Autodesk Fusion 360 part; units mm, degrees
note: some values were not read from the file. Chosen so that the rebuilt part matches the saved one: which bodies a step acts on; which face or edge a step refers to; where a step ends.
(part 2 of 2)
sketch "Sketch2 (3)" plane through (-245, 0, 0) normal (-1, 0, 0) x (0, 0, 1) in component "Обшивка-Плиты"
  line L0 (-212.9492, 20) -> (-218.3368, 15)
  line L1 (-218.3368, 15) -> (0, 15)
  line L2 (0, 15) -> (0, 20)
  line L3 (0, 20) -> (-212.9492, 20)
  line L4 (-500, 15) -> (-250, 15)
  line L5 (-250, 15) -> (-250, 140)
  line L6 (-250, 140) -> (-500, 140)
  line L7 (-500, 140) -> (-500, 15)
  line L8 (-500, 140) -> (-250, 140)
  line L9 (-250, 140) -> (-250, 265)
  line L10 (-250, 265) -> (-500, 265)
  line L11 (-500, 265) -> (-500, 140)
  line L12 (-250, 15) -> (0, 15)
  line L13 (0, 15) -> (0, 140)
  line L14 (0, 140) -> (-250, 140)
  line L15 (-250, 140) -> (-250, 15)
  line L16 (-250, 140) -> (0, 140)
  line L17 (0, 140) -> (0, 265)
  line L18 (0, 265) -> (-250, 265)
  line L19 (-250, 265) -> (-250, 140)
  point P0 (-500, 15)
  dimension "d244" = 250
  dimension "d245" = 125
  dimension "d246" = 250
  dimension "d247" = 125
  dimension "d248" = 250
  dimension "d249" = 125
  dimension "d250" = 250
  dimension "d251" = 125
  constraint horizontal L4
  constraint vertical L5
  constraint horizontal L6
  constraint vertical L7
  constraint coincident P0 L4.start
  constraint horizontal L8
  constraint vertical L9
  constraint horizontal L10
  constraint vertical L11
  constraint horizontal L12
  constraint vertical L13
  constraint horizontal L14
  constraint vertical L15
  constraint horizontal L16
  constraint vertical L17
  constraint horizontal L18
  constraint vertical L19
  measures "d244" distance of P0 L4.end
  measures "d245" distance of P0 L6.end
  measures "d246" distance of L6.end L5.end
  measures "d247" distance of L6.end L10.end
  measures "d248" distance of L4.end L1.end
  measures "d249" distance of L4.end L5.end
  measures "d250" distance of L5.end L13.end
  measures "d251" distance of L5.end L9.end
extrude "Extrude6''" add sketch "Sketch2 (3)" along normal blind 1.12 separate body contours L4 L5 L6 L7 L8 L15 makes body 113 in component "Обшивка-Плиты"
extrude "Extrude7" add sketch "Sketch2 (3)" along normal blind 1.12 separate body contours L6 L8 L9 L10 L11 L19 makes body 114 in component "Обшивка-Плиты"
extrude "Extrude8" add sketch "Sketch2 (3)" along normal blind 1.12 separate body contours L9 L14 L16 L17 L18 L19 makes body 115 in component "Обшивка-Плиты"
extrude "Extrude9" add sketch "Sketch2 (3)" along normal blind 1.12 separate body contours L0 L1 L2 L3 L12 L13 | L0 L3 L5 L12 L13 L14 L15 L16 makes body 116 in component "Обшивка-Плиты"
split "Split1" by plane through (-259.4882, 213.5887, -495) normal (-0.190809, 0.981627, 0) bodies 114 115 makes body 118 at (-246.12, 232.4581, -83.3333) makes body 117 at (-246.12, 232.4581, -333.3333) in component "Обшивка-Плиты"
delete_body "RemoveBody1" bodies 118 in component "Обшивка-Плиты"
delete_body "RemoveBody2" bodies 117 in component "Обшивка-Плиты"
combine "Combine5'" operation cut target body 114 tool bodies 79 78 77 76 75 keep tools in component "Обшивка-Плиты"
combine "Combine6'" operation cut target body 115 tool bodies 74 73 72 71 keep tools in component "Обшивка-Плиты"
sketch "Sketch3 (3)" plane through (0, 0, 0) normal (0, 0, 1) x (1, 0, 0) in component "Обшивка-Плиты"
  line L0 (-194.3541, 20) -> (-199.0829, 15)
  line L1 (-199.0829, 15) -> (-5, 15)
  line L2 (-5, 15) -> (-5, 20)
  line L3 (-5, 20) -> (-194.3541, 20)
  line L4 (-245, 15) -> (5, 15)
  line L5 (5, 15) -> (5, 140)
  line L6 (5, 140) -> (-245, 140)
  line L7 (-245, 140) -> (-245, 15)
  line L8 (-245, 140) -> (5, 140)
  line L9 (5, 140) -> (5, 265)
  line L10 (5, 265) -> (-245, 265)
  line L11 (-245, 265) -> (-245, 140)
  point P0 (-245, 15)
  dimension "d260" = 250
  dimension "d261" = 125
  dimension "d262" = 250
  dimension "d263" = 125
  constraint horizontal L4
  constraint vertical L5
  constraint horizontal L6
  constraint vertical L7
  constraint coincident P0 L4.start
  constraint horizontal L8
  constraint vertical L9
  constraint horizontal L10
  constraint vertical L11
  measures "d260" distance of P0 L4.end
  measures "d261" distance of P0 L6.end
  measures "d262" distance of L6.end L5.end
  measures "d263" distance of L6.end L10.end
extrude "Extrude10" add sketch "Sketch3 (3)" along normal blind 1.12 separate body contours L0 L1 L2 L3 L4 | L0 L2 L3 L4 L5 L6 L7 L8 makes body 119 in component "Обшивка-Плиты"
extrude "Extrude11" add sketch "Sketch3 (3)" along normal blind 1.12 separate body contours L6 L8 L9 L10 L11 makes body 120 in component "Обшивка-Плиты"
split "Split2" by plane through (-259.4882, 213.5887, 0) normal (-0.190809, 0.981627, 0) bodies 120 makes body 121 at (-161.6667, 248.8016, 0) in component "Обшивка-Плиты"
delete_body "RemoveBody3" bodies 121 in component "Обшивка-Плиты"
mirror "Mirror1" about plane through (0, 0, -250) normal (0, 0, 1) of bodies 119 120 makes body 122 at (-146.361, 98.3333, -500) makes body 123 at (-78.3333, 207.135, -500) in component "Обшивка-Плиты"
extrude "Extrude12" add sketch "Sketch1 (9)" along normal blind 1.12 separate body contours L5 L13 L16 L17 L18 L19 makes body 124 in component "Обшивка-Плиты"
combine "Combine7'" operation cut target body 124 tool bodies 74 keep tools in component "Обшивка-Плиты"
sketch "Sketch1 (10)" plane through (5, 0, 0) normal (1, 0, 0) x (0, 0, -1) in component "Обшивка-Доски"
  line L0 (270.8891, 15) -> (275, 20)
  line L1 (275, 20) -> (0, 20)
  line L2 (0, 20) -> (0, 15)
  line L3 (0, 15) -> (270.8891, 15)
  line L4 (0, 15) -> (125, 15)
  line L5 (125, 15) -> (125, 30)
  line L6 (125, 30) -> (0, 30)
  line L7 (0, 30) -> (0, 15)
  point P0 (0, 15)
  dimension "d273" = 125
  dimension "d274" = 15
  constraint horizontal L4
  constraint vertical L5
  constraint horizontal L6
  constraint vertical L7
  constraint coincident P0 L2.end
  measures "d273" distance of P0 L4.end
  measures "d274" distance of P0 L6.end
extrude "Extrude1'''''''''" add sketch "Sketch1 (10)" along normal blind 1 separate body contours L1 L2 L3 L4 L5 L7 | L1 L5 L6 L7 makes body 125 in component "Обшивка-Доски"
pattern_linear "R-Pattern1''''''" count 17 spacing 15 along (0, 1, 0) of bodies 125 makes body 126 at (5, 38.3333, -41.6667) makes body 127 at (5, 53.3333, -41.6667) makes body 128 at (5, 68.3333, -41.6667) makes body 129 at (5, 83.3333, -41.6667) makes body 130 at (5, 98.3333, -41.6667) makes body 131 at (5, 113.3333, -41.6667) makes body 132 at (5, 128.3333, -41.6667) makes body 133 at (5, 143.3333, -41.6667) makes body 134 at (5, 158.3333, -41.6667) makes body 135 at (5, 173.3333, -41.6667) makes body 136 at (5, 188.3333, -41.6667) makes body 137 at (5, 203.3333, -41.6667) makes body 138 at (5, 218.3333, -41.6667) makes body 139 at (5, 233.3333, -41.6667) makes body 140 at (5, 248.3333, -41.6667) makes body 141 at (5, 263.3333, -41.6667) in component "Обшивка-Доски"
split "Split1'" by plane through (230.3104, 308.7959, 0) normal (0.190809, -0.981627, 0) bodies 141 makes body 142 at (6, 263.4629, -41.6667) in component "Обшивка-Доски"
delete_body "RemoveBody1'" bodies 141 in component "Обшивка-Доски"
copy_body "CopyPasteBodies1'''''" bodies 138 139 140 142 makes body 143 makes body 144 makes body 145 makes body 146
move_body "Move1'''''''" bodies 143 144 145 146 to x (1, 0, 0) y (0, 1, 0) z (0, 0, 1) at (0, 0, -125)
delete_body "RemoveBody1''" bodies 143
delete_body "RemoveBody2'" bodies 146
delete_body "RemoveBody3'" bodies 145
delete_body "RemoveBody4'" bodies 144
copy_body "CopyPasteBodies1''''''" bodies 142 140 139 138 makes body 147 makes body 148 makes body 149 makes body 150 in component "Обшивка-Доски"
move_body "Move1''''''''" bodies 147 148 149 150 to x (1, 0, 0) y (0, 1, 0) z (0, 0, 1) at (0, 0, -125) in component "Обшивка-Доски"
copy_body "CopyPasteBodies2''''''" bodies 142 126 125 127 128 129 130 131 137 138 140 135 139 136 134 133 132 makes body 151 makes body 152 makes body 153 makes body 154 makes body 155 makes body 156 makes body 157 makes body 158 makes body 159 makes body 160 makes body 161 makes body 162 makes body 163 makes body 164 makes body 165 makes body 166 makes body 167 in component "Обшивка-Доски"
move_body "Move2''''''''" bodies 151 152 153 154 155 156 157 158 159 160 161 162 163 164 165 166 167 to x (1, 0, 0) y (0, 1, 0) z (0, 0, 1) at (0, 0, -250) in component "Обшивка-Доски"
copy_body "CopyPasteBodies3''''''" bodies 142 126 125 127 128 129 130 131 137 138 140 135 139 136 134 133 132 makes body 168 makes body 169 makes body 170 makes body 171 makes body 172 makes body 173 makes body 174 makes body 175 makes body 176 makes body 177 makes body 178 makes body 179 makes body 180 makes body 181 makes body 182 makes body 183 makes body 184 in component "Обшивка-Доски"
move_body "Move3'''''''" bodies 168 169 170 171 172 173 174 175 176 177 178 179 180 181 182 183 184 to x (1, 0, 0) y (0, 1, 0) z (0, 0, 1) at (0, 0, -375) in component "Обшивка-Доски"
combine "Combine1''" operation cut target body 142 tool bodies 71 72 73 keep tools makes body 185 at (6, 261.7963, -84.5833) in component "Обшивка-Доски"
combine "Combine2''" operation cut target body 140 tool bodies 71 72 73 keep tools in component "Обшивка-Доски"
combine "Combine3''" operation cut target body 147 tool bodies 74 keep tools makes body 186 at (6, 258.3981, -210.4167) in component "Обшивка-Доски"
combine "Combine4''" operation cut target body 148 tool bodies 74 keep tools in component "Обшивка-Доски"
combine "Combine5''" operation cut target body 151 tool bodies 75 76 77 keep tools makes body 187 at (6, 261.7963, -333.3333) in component "Обшивка-Доски"
combine "Combine6''" operation cut target body 161 tool bodies 75 76 77 keep tools in component "Обшивка-Доски"
combine "Combine7''" operation cut target body 168 tool bodies 78 79 keep tools makes body 188 at (6, 261.7963, -413.75) in component "Обшивка-Доски"
combine "Combine8'" operation cut target body 178 tool bodies 78 79 keep tools in component "Обшивка-Доски"
sketch "Sketch2 (4)" plane through (0, 0, 0) normal (0, 0, 1) x (1, 0, 0) in component "Обшивка-Доски"
  line L0 (-194.3541, 20) -> (-199.0829, 15)
  line L1 (-199.0829, 15) -> (-5, 15)
  line L2 (-5, 15) -> (-5, 20)
  line L3 (-5, 20) -> (-194.3541, 20)
  line L4 (-245, 15) -> (5, 15)
  line L5 (5, 15) -> (5, 30)
  line L6 (5, 30) -> (-245, 30)
  line L7 (-245, 30) -> (-245, 15)
  point P0 (-245, 15)
  point P1 (5, 15)
  dimension "d281" = 250
  dimension "d282" = 15
  constraint horizontal L4
  constraint vertical L5
  constraint horizontal L6
  constraint vertical L7
  constraint coincident P0 L4.start
  measures "d281" distance of P0 P1
  measures "d282" distance of P0 L6.end
extrude "Extrude2''''" add sketch "Sketch2 (4)" along normal blind 1 separate body makes body 189 in component "Обшивка-Доски"
pattern_linear "R-Pattern2" count 17 spacing 15 along (0, 1, 0) of bodies 189 makes body 190 at (-146.361, 40, 0) makes body 191 at (-146.361, 55, 0) makes body 192 at (-146.361, 70, 0) makes body 193 at (-146.361, 85, 0) makes body 194 at (-146.361, 100, 0) makes body 195 at (-146.361, 115, 0) makes body 196 at (-146.361, 130, 0) makes body 197 at (-146.361, 145, 0) makes body 198 at (-146.361, 160, 0) makes body 199 at (-146.361, 175, 0) makes body 200 at (-146.361, 190, 0) makes body 201 at (-146.361, 205, 0) makes body 202 at (-146.361, 220, 0) makes body 203 at (-146.361, 235, 0) makes body 204 at (-146.361, 250, 0) makes body 205 at (-146.361, 265, 0) in component "Обшивка-Доски"
split "Split2'" by plane through (-259.4882, 213.5887, 0) normal (-0.190809, 0.981627, 0) bodies 205 204 203 202 makes body 209 at (-230.2607, 222.135, 0) makes body 208 at (-189.7987, 235, 0) makes body 207 at (-138.3531, 250, 0) makes body 206 at (-95.4818, 265, 0) in component "Обшивка-Доски"
delete_body "RemoveBody2''" bodies 209 in component "Обшивка-Доски"
delete_body "RemoveBody3''" bodies 208 in component "Обшивка-Доски"
delete_body "RemoveBody4''" bodies 207 in component "Обшивка-Доски"
delete_body "RemoveBody5" bodies 206 in component "Обшивка-Доски"
mirror "Mirror1'" about plane through (0, 0, -250) normal (0, 0, 1) of bodies 189 198 203 190 195 200 199 192 204 194 205 201 191 197 202 193 196 makes body 210 at (-146.361, 25, -500) makes body 211 at (-146.361, 40, -500) makes body 212 at (-146.361, 55, -500) makes body 213 at (-146.361, 70, -500) makes body 214 at (-146.361, 85, -500) makes body 215 at (-146.361, 100, -500) makes body 216 at (-146.361, 115, -500) makes body 217 at (-146.361, 130, -500) makes body 218 at (-146.361, 145, -500) makes body 219 at (-146.361, 160, -500) makes body 220 at (-146.361, 175, -500) makes body 221 at (-146.361, 190, -500) makes body 222 at (-146.361, 205, -500) makes body 223 at (-66.9274, 220, -500) makes body 224 at (-109.2323, 230, -500) makes body 225 at (-58.3531, 245, -500) makes body 226 at (-15.4818, 258.3333, -500) in component "Обшивка-Доски"
sketch "Sketch3 (4)" plane through (-245, 0, 0) normal (-1, 0, 0) x (0, 0, 1) in component "Обшивка-Доски"
  line L0 (-36.6632, 204.068) -> (-240.3876, 15)
  line L1 (-240.3876, 15) -> (-218.3368, 15)
  line L2 (-218.3368, 15) -> (-14.6124, 204.068)
  line L3 (-14.6124, 204.068) -> (-36.6632, 204.068)
  line L4 (-500, 15) -> (0, 15)
  line L5 (0, 15) -> (0, 30)
  line L6 (0, 30) -> (-500, 30)
  line L7 (-500, 30) -> (-500, 15)
  point P0 (-500, 15)
  dimension "d291" = 500
  dimension "d292" = 15
  constraint horizontal L4
  constraint vertical L5
  constraint horizontal L6
  constraint vertical L7
  constraint coincident P0 L4.start
  measures "d291" distance of P0 L4.end
  measures "d292" distance of P0 L6.end
extrude "Extrude3''''" add sketch "Sketch3 (4)" along normal blind 1 separate body contours L0 L1 L2 L4 L6 | L0 L4 L6 L7 | L2 L4 L5 L6 makes body 227 in component "Обшивка-Доски"
pattern_linear "R-Pattern3" count 13 spacing 15 along (0, 1, 0) of bodies 227 makes body 228 at (-245, 40, -321.5375) makes body 229 at (-245, 55, -321.5375) makes body 230 at (-245, 70, -321.5375) makes body 231 at (-245, 85, -321.5375) makes body 232 at (-245, 100, -321.5375) makes body 233 at (-245, 115, -321.5375) makes body 234 at (-245, 130, -321.5375) makes body 235 at (-245, 145, -321.5375) makes body 236 at (-245, 160, -321.5375) makes body 237 at (-245, 175, -321.5375) makes body 238 at (-245, 190, -321.5375) makes body 239 at (-245, 205, -321.5375) in component "Обшивка-Доски"
sketch "Sketch3 (5)" plane through (0, 0, 0) normal (0, 0, 1) x (1, 0, 0) in component "Стропила"
  line L0 (5, 250.7192) -> (5, 249.7192)
  line L1 (5, 249.7192) -> (35, 255.5507)
  line L2 (35, 255.5507) -> (35, 270.8314)
  line L3 (35, 270.8314) -> (-259.4882, 213.5887)
  line L4 (-259.4882, 213.5887) -> (-256.626, 198.8643)
  line L5 (-256.626, 198.8643) -> (-245, 201.1242)
  line L6 (-245, 201.1242) -> (-245, 204.068)
  line L7 (-245, 204.068) -> (-229.8554, 204.068)
  line L8 (-229.8554, 204.068) -> (-5, 247.7754)
  line L9 (-5, 247.7754) -> (-5, 250.7192)
  line L10 (-5, 250.7192) -> (5, 250.7192)
  line L11 (-256.626, 198.8643) -> (-259.4882, 213.5887)
  line L12 (-259.4882, 213.5887) -> (-257.0341, 214.0657)
  line L13 (-257.0341, 214.0657) -> (-254.172, 199.3413)
  line L14 (-254.172, 199.3413) -> (-256.626, 198.8643)
  line L15 (35, 255.5507) -> (32.5, 255.5507)
  line L16 (32.5, 255.5507) -> (32.5, 270.5507)
  line L17 (32.5, 270.5507) -> (35, 270.5507)
  line L18 (35, 270.5507) -> (35, 255.5507)
  dimension "d299" = 2.5
  dimension "d300" = 2.5
  dimension "d301" = 15
  constraint perpendicular L11 L12
  constraint parallel L11 L13
  constraint parallel L12 L14
  constraint coincident L3.end L4.start
  constraint perpendicular L3 L11
  constraint coincident L4.end L5.start
  constraint horizontal L15
  constraint vertical L16
  constraint horizontal L17
  constraint vertical L18
  constraint coincident L1.end L2.start
  measures "d299" distance of L4.end L13.end
  measures "d300" distance of L1.end L15.end
  measures "d301" distance of L1.end L17.end
extrude "Extrude2'''''" add sketch "Sketch3 (5)" against normal blind 500 separate body contours L2 L3 L15 L16 L17 L18 makes body 240 in component "Стропила"
extrude "Extrude3'''''" add sketch "Sketch3 (5)" against normal blind 500 separate body contours L3 L4 L5 L11 L12 L13 L14 makes body 241 in component "Стропила"
combine "Combine12" operation cut target body 71 tool bodies 241 keep tools in component "Стропила"
combine "Combine13" operation cut target body 72 tool bodies 241 keep tools in component "Стропила"
combine "Combine14" operation cut target body 73 tool bodies 241 keep tools in component "Стропила"
combine "Combine15" operation cut target body 74 tool bodies 241 keep tools in component "Стропила"
combine "Combine16" operation cut target body 75 tool bodies 241 keep tools in component "Стропила"
combine "Combine17" operation cut target body 76 tool bodies 241 keep tools in component "Стропила"
combine "Combine18" operation cut target body 77 tool bodies 241 keep tools in component "Стропила"
combine "Combine19" operation cut target body 78 tool bodies 241 keep tools in component "Стропила"
combine "Combine20" operation cut target body 79 tool bodies 241 keep tools in component "Стропила"
split "Split1''" by plane through (32.5, 255.5507, 0) normal (1, 0, 0) bodies 71 78 76 79 75 77 73 72 74 makes body 250 at (-165.678, 222.951, -185.625) makes body 249 at (-165.678, 222.951, -61.875) makes body 248 at (-165.678, 222.951, -120) makes body 247 at (-165.678, 222.951, -371.25) makes body 246 at (-165.678, 222.951, -250) makes body 245 at (-163.9632, 222.951, -495) makes body 244 at (-165.678, 222.951, -309.375) makes body 243 at (-165.678, 222.951, -433.125) makes body 242 at (-163.9632, 222.951, 0) in component "Стропила"
delete_body "RemoveBody1'''" bodies 79 in component "Стропила"
delete_body "RemoveBody2'''" bodies 78 in component "Стропила"
delete_body "RemoveBody3'''" bodies 76 in component "Стропила"
delete_body "RemoveBody4'''" bodies 75 in component "Стропила"
delete_body "RemoveBody5'" bodies 77 in component "Стропила"
delete_body "RemoveBody6" bodies 73 in component "Стропила"
delete_body "RemoveBody7" bodies 72 in component "Стропила"
delete_body "RemoveBody8" bodies 74 in component "Стропила"
delete_body "RemoveBody9" bodies 71 in component "Стропила"
sketch "Sketch1 (11)" plane through (5, 0, 0) normal (1, 0, 0) x (0, 0, -1) in component "Обшивка-Доски-Вертикально"
  line L0 (270.8891, 15) -> (275, 20)
  line L1 (275, 20) -> (0, 20)
  line L2 (0, 20) -> (0, 15)
  line L3 (0, 15) -> (270.8891, 15)
  line L4 (0, 15) -> (15, 15)
  line L5 (15, 15) -> (15, 315)
  line L6 (15, 315) -> (0, 315)
  line L7 (0, 315) -> (0, 15)
  dimension "d306" = 15
  dimension "d307" = 300
  constraint horizontal L4
  constraint vertical L5
  constraint horizontal L6
  constraint vertical L7
  constraint coincident L2.end L3.start
  measures "d306" distance of L2.end L4.end
  measures "d307" distance of L2.end L6.end
extrude "Extrude1''''''''''" add sketch "Sketch1 (11)" along normal blind 1 separate body contours L1 L2 L3 L4 L5 L7 | L1 L5 L6 L7 makes body 251 in component "Обшивка-Доски-Вертикально"
split "Split1'''" by bodies 96 bodies 251 makes body 252 at (5, 216.6667, -5) in component "Обшивка-Доски-Вертикально"
delete_body "RemoveBody1''''" bodies 251 in component "Обшивка-Доски-Вертикально"
split "Split2''" by plane through (230.3104, 308.7959, 0) normal (0.190809, -0.981627, 0) bodies 252 makes body 253 at (6, 101.7315, -5) in component "Обшивка-Доски-Вертикально"
delete_body "RemoveBody2''''" bodies 252 in component "Обшивка-Доски-Вертикально"
pattern_linear "R-Pattern1'''''''" count 33 spacing 15.1562 along (0, 0, -1) of bodies 253 makes body 254 at (6, 101.7315, -20.1562) makes body 255 at (6, 101.7315, -35.3125) makes body 256 at (6, 101.7315, -50.4688) makes body 257 at (6, 101.7315, -65.625) makes body 258 at (6, 101.7315, -80.7812) makes body 259 at (6, 101.7315, -95.9375) makes body 260 at (6, 101.7315, -111.0938) makes body 261 at (6, 101.7315, -126.25) makes body 262 at (6, 101.7315, -141.4062) makes body 263 at (6, 101.7315, -156.5625) makes body 264 at (6, 101.7315, -171.7188) makes body 265 at (6, 101.7315, -186.875) makes body 266 at (6, 101.7315, -202.0312) makes body 267 at (6, 101.7315, -217.1875) makes body 268 at (6, 101.7315, -232.3438) makes body 269 at (6, 101.7315, -247.5) makes body 270 at (6, 101.7315, -262.6562) makes body 271 at (6, 101.7315, -277.8125) makes body 272 at (6, 101.7315, -292.9688) makes body 273 at (6, 101.7315, -308.125) makes body 274 at (6, 101.7315, -323.2812) makes body 275 at (6, 101.7315, -338.4375) makes body 276 at (6, 101.7315, -353.5938) makes body 277 at (6, 101.7315, -368.75) makes body 278 at (6, 101.7315, -383.9062) makes body 279 at (6, 101.7315, -399.0625) makes body 280 at (6, 101.7315, -414.2188) makes body 281 at (6, 101.7315, -429.375) makes body 282 at (6, 101.7315, -444.5312) makes body 283 at (6, 101.7315, -459.6875) makes body 284 at (6, 101.7315, -474.8438) makes body 285 at (6, 101.7315, -490) in component "Обшивка-Доски-Вертикально"
split "Split3" by plane through (-5, 210.0714, -120) normal (0, -1, 0) bodies 261 262 263 264 265 266 267 268 269 makes body 294 at (5, 146.7143, -247.5) makes body 293 at (5, 146.7143, -232.3438) makes body 292 at (5, 146.7143, -217.1875) makes body 291 at (5, 146.7143, -202.0312) makes body 290 at (5, 146.7143, -186.875) makes body 289 at (5, 146.7143, -171.7188) makes body 288 at (5, 146.7143, -156.5625) makes body 287 at (5, 146.7143, -141.4062) makes body 286 at (5, 146.7143, -126.25) in component "Обшивка-Доски-Вертикально"
delete_body "RemoveBody3''''" bodies 293 in component "Обшивка-Доски-Вертикально"
delete_body "RemoveBody4''''" bodies 289 in component "Обшивка-Доски-Вертикально"
delete_body "RemoveBody5''" bodies 288 in component "Обшивка-Доски-Вертикально"
delete_body "RemoveBody6'" bodies 290 in component "Обшивка-Доски-Вертикально"
delete_body "RemoveBody7'" bodies 287 in component "Обшивка-Доски-Вертикально"
delete_body "RemoveBody8'" bodies 291 in component "Обшивка-Доски-Вертикально"
delete_body "RemoveBody9'" bodies 292 in component "Обшивка-Доски-Вертикально"
combine "Combine1'''" operation add target body 286 tool bodies 261 keep tools in component "Обшивка-Доски-Вертикально"
combine "Combine2'''" operation add target body 294 tool bodies 269 keep tools in component "Обшивка-Доски-Вертикально"
delete_body "RemoveBody10" bodies 261 in component "Обшивка-Доски-Вертикально"
delete_body "RemoveBody11" bodies 269 in component "Обшивка-Доски-Вертикально"
split "Split4" by plane through (-5, 210.0714, -120) normal (0, -1, 0) bodies 294 makes body 295 at (5, 80.0238, -247.5) in component "Обшивка-Доски-Вертикально"
split "Split5" by plane through (0, 0, -250) normal (0, 0, 1) bodies 295 makes body 296 at (5, 80.0238, -245) in component "Обшивка-Доски-Вертикально"
delete_body "RemoveBody12" bodies 296 in component "Обшивка-Доски-Вертикально"
combine "Combine3'''" operation add target body 294 tool bodies 295 in component "Обшивка-Доски-Вертикально"
split "Split6" by plane through (-5, 210.0714, -120) normal (0, -1, 0) bodies 286 makes body 297 at (5, 80.0238, -126.25) in component "Обшивка-Доски-Вертикально"
split "Split7" by plane through (0, 0, -125) normal (0, 0, -1) bodies 297 makes body 298 at (5, 80.0238, -128.75) in component "Обшивка-Доски-Вертикально"
delete_body "RemoveBody13" bodies 298 in component "Обшивка-Доски-Вертикально"
combine "Combine4'''" operation add target body 297 tool bodies 286 in component "Обшивка-Доски-Вертикально"
sketch "Sketch2 (5)" plane through (0, 0, 0) normal (0, 0, 1) x (1, 0, 0) in component "Обшивка-Доски-Вертикально"
  line L0 (-219.7288, 15) -> (-199.0829, 15)
  line L1 (-199.0829, 15) -> (-20.2712, 204.068)
  line L2 (-20.2712, 204.068) -> (-40.9171, 204.068)
  line L3 (-40.9171, 204.068) -> (-219.7288, 15)
  line L4 (5, 15) -> (-10, 15)
  line L5 (-10, 15) -> (-10, 265)
  line L6 (-10, 265) -> (5, 265)
  line L7 (5, 265) -> (5, 15)
  point P0 (5, 15)
  dimension "d314" = 15
  dimension "d315" = 250
  constraint horizontal L4
  constraint vertical L5
  constraint horizontal L6
  constraint vertical L7
  constraint coincident P0 L4.start
  measures "d314" distance of P0 L4.end
  measures "d315" distance of P0 L6.end
extrude "Extrude2''''''" add sketch "Sketch2 (5)" along normal blind 1 separate body contours L4 L5 L6 L7 makes body 299 in component "Обшивка-Доски-Вертикально"
pattern_linear "R-Pattern2'" count 16 spacing 15.6667 along (-1, 0, 0) of bodies 299 makes body 300 at (-15.6667, 98.3333, 0) makes body 301 at (-31.3333, 98.3333, 0) makes body 302 at (-47, 98.3333, 0) makes body 303 at (-62.6667, 98.3333, 0) makes body 304 at (-78.3333, 98.3333, 0) makes body 305 at (-94, 98.3333, 0) makes body 306 at (-109.6667, 98.3333, 0) makes body 307 at (-125.3333, 98.3333, 0) makes body 308 at (-141, 98.3333, 0) makes body 309 at (-156.6667, 98.3333, 0) makes body 310 at (-172.3333, 98.3333, 0) makes body 311 at (-188, 98.3333, 0) makes body 312 at (-203.6667, 98.3333, 0) makes body 313 at (-219.3333, 98.3333, 0) makes body 314 at (-235, 98.3333, 0) in component "Обшивка-Доски-Вертикально"
split "Split8" by plane through (-259.4882, 213.5887, 0) normal (-0.190809, 0.981627, 0) bodies 299 300 308 307 309 306 310 312 313 314 311 305 301 302 303 304 makes body 330 at (-83.3333, 253.8771, 0) makes body 329 at (-67.6667, 255.9073, 0) makes body 328 at (-52, 257.9375, 0) makes body 327 at (-36.3333, 259.9677, 0) makes body 326 at (-99, 251.8469, 0) makes body 325 at (-193, 239.6658, 0) makes body 324 at (-240, 233.5752, 0) makes body 323 at (-224.3333, 235.6054, 0) makes body 322 at (-208.6667, 237.6356, 0) makes body 321 at (-177.3333, 241.696, 0) makes body 320 at (-114.6667, 249.8167, 0) makes body 319 at (-161.6667, 243.7262, 0) makes body 318 at (-130.3333, 247.7865, 0) makes body 317 at (-146, 245.7563, 0) makes body 316 at (-20.6667, 261.9979, 0) makes body 315 at (-5, 264.0281, 0) in component "Обшивка-Доски-Вертикально"
delete_body "RemoveBody14" bodies 315 in component "Обшивка-Доски-Вертикально"
delete_body "RemoveBody15" bodies 327 in component "Обшивка-Доски-Вертикально"
delete_body "RemoveBody16" bodies 326 in component "Обшивка-Доски-Вертикально"
delete_body "RemoveBody17" bodies 318 in component "Обшивка-Доски-Вертикально"
delete_body "RemoveBody18" bodies 320 in component "Обшивка-Доски-Вертикально"
delete_body "RemoveBody19" bodies 319 in component "Обшивка-Доски-Вертикально"
delete_body "RemoveBody20" bodies 317 in component "Обшивка-Доски-Вертикально"
delete_body "RemoveBody21" bodies 316 in component "Обшивка-Доски-Вертикально"
delete_body "RemoveBody22" bodies 321 in component "Обшивка-Доски-Вертикально"
delete_body "RemoveBody23" bodies 322 in component "Обшивка-Доски-Вертикально"
delete_body "RemoveBody24" bodies 325 in component "Обшивка-Доски-Вертикально"
delete_body "RemoveBody25" bodies 324 in component "Обшивка-Доски-Вертикально"
delete_body "RemoveBody26" bodies 323 in component "Обшивка-Доски-Вертикально"
delete_body "RemoveBody27" bodies 328 in component "Обшивка-Доски-Вертикально"
delete_body "RemoveBody28" bodies 330 in component "Обшивка-Доски-Вертикально"
delete_body "RemoveBody29" bodies 329 in component "Обшивка-Доски-Вертикально"
mirror "Mirror1''" about plane through (0, 0, -250) normal (0, 0, 1) of bodies 299 300 308 307 309 306 310 312 313 314 311 305 301 302 303 304 makes body 331 at (0, 180.6948, -500) makes body 332 at (-15.6667, 178.6646, -500) makes body 333 at (-31.3333, 176.6344, -500) makes body 334 at (-47, 174.6042, -500) makes body 335 at (-62.6667, 172.574, -500) makes body 336 at (-78.3333, 170.5438, -500) makes body 337 at (-94, 168.5136, -500) makes body 338 at (-109.6667, 166.4834, -500) makes body 339 at (-125.3333, 164.4532, -500) makes body 340 at (-141, 162.423, -500) makes body 341 at (-156.6667, 160.3928, -500) makes body 342 at (-172.3333, 158.3626, -500) makes body 343 at (-188, 156.3324, -500) makes body 344 at (-203.6667, 154.3022, -500) makes body 345 at (-219.3333, 152.272, -500) makes body 346 at (-235, 150.2419, -500) in component "Обшивка-Доски-Вертикально"
sketch "Sketch3 (6)" plane through (-245, 0, 0) normal (-1, 0, 0) x (0, 0, 1) in component "Обшивка-Доски-Вертикально"
  line L0 (-286.5071, 15) -> (-291.7631, 20)
  line L1 (-291.7631, 20) -> (-500, 20)
  line L2 (-500, 20) -> (-500, 15)
  line L3 (-500, 15) -> (-286.5071, 15)
  line L4 (0, 15) -> (-15, 15)
  line L5 (-15, 15) -> (-15, 265)
  line L6 (-15, 265) -> (0, 265)
  line L7 (0, 265) -> (0, 15)
  point P0 (0, 15)
  dimension "d324" = 15
  dimension "d325" = 250
  constraint horizontal L4
  constraint vertical L5
  constraint horizontal L6
  constraint vertical L7
  constraint coincident P0 L4.start
  measures "d324" distance of P0 L4.end
  measures "d325" distance of P0 L6.end
extrude "Extrude3''''''" add sketch "Sketch3 (6)" along normal blind 1 separate body contours L4 L5 L6 L7 makes body 347 in component "Обшивка-Доски-Вертикально"
pattern_linear "R-Pattern3'" count 33 spacing 15.1562 along (0, 0, -1) of bodies 347 makes body 348 at (-245, 98.3333, -20.1562) makes body 349 at (-245, 98.3333, -35.3125) makes body 350 at (-245, 98.3333, -50.4688) makes body 351 at (-245, 98.3333, -65.625) makes body 352 at (-245, 98.3333, -80.7812) makes body 353 at (-245, 98.3333, -95.9375) makes body 354 at (-245, 98.3333, -111.0938) makes body 355 at (-245, 98.3333, -126.25) makes body 356 at (-245, 98.3333, -141.4062) makes body 357 at (-245, 98.3333, -156.5625) makes body 358 at (-245, 98.3333, -171.7188) makes body 359 at (-245, 98.3333, -186.875) makes body 360 at (-245, 98.3333, -202.0312) makes body 361 at (-245, 98.3333, -217.1875) makes body 362 at (-245, 98.3333, -232.3438) makes body 363 at (-245, 98.3333, -247.5) makes body 364 at (-245, 98.3333, -262.6562) makes body 365 at (-245, 98.3333, -277.8125) makes body 366 at (-245, 98.3333, -292.9688) makes body 367 at (-245, 98.3333, -308.125) makes body 368 at (-245, 98.3333, -323.2812) makes body 369 at (-245, 98.3333, -338.4375) makes body 370 at (-245, 98.3333, -353.5938) makes body 371 at (-245, 98.3333, -368.75) makes body 372 at (-245, 98.3333, -383.9062) makes body 373 at (-245, 98.3333, -399.0625) makes body 374 at (-245, 98.3333, -414.2188) makes body 375 at (-245, 98.3333, -429.375) makes body 376 at (-245, 98.3333, -444.5312) makes body 377 at (-245, 98.3333, -459.6875) makes body 378 at (-245, 98.3333, -474.8438) makes body 379 at (-245, 98.3333, -490) in component "Обшивка-Доски-Вертикально"
split "Split9" by plane through (-259.4882, 213.5887, 0) normal (-0.190809, 0.981627, 0) bodies 347 368 367 353 351 352 350 349 362 361 363 348 364 365 359 366 360 369 373 375 376 372 374 377 378 379 370 371 358 356 355 354 357 makes body 412 at (-246, 232.4737, -156.5625) makes body 411 at (-246, 232.4737, -111.0938) makes body 410 at (-246, 232.4737, -126.25) makes body 409 at (-246, 232.4737, -141.4062) makes body 408 at (-246, 232.4737, -171.7188) makes body 407 at (-246, 232.4737, -368.75) makes body 406 at (-246, 232.4737, -353.5938) makes body 405 at (-246, 232.4737, -490) makes body 404 at (-246, 232.4737, -474.8438) makes body 403 at (-246, 232.4737, -459.6875) makes body 402 at (-246, 232.4737, -414.2188) makes body 401 at (-246, 232.4737, -383.9062) makes body 400 at (-246, 232.4737, -444.5312) makes body 399 at (-246, 232.4737, -429.375) makes body 398 at (-246, 232.4737, -399.0625) makes body 397 at (-246, 232.4737, -338.4375) makes body 396 at (-246, 232.4737, -202.0312) makes body 395 at (-246, 232.4737, -292.9688) makes body 394 at (-246, 232.4737, -186.875) makes body 393 at (-246, 232.4737, -277.8125) makes body 392 at (-246, 232.4737, -262.6562) makes body 391 at (-246, 232.4737, -20.1562) makes body 390 at (-246, 232.4737, -247.5) makes body 389 at (-246, 232.4737, -217.1875) makes body 388 at (-246, 232.4737, -232.3438) makes body 387 at (-246, 232.4737, -35.3125) makes body 386 at (-246, 232.4737, -50.4688) makes body 385 at (-246, 232.4737, -80.7812) makes body 384 at (-246, 232.4737, -65.625) makes body 383 at (-246, 232.4737, -95.9375) makes body 382 at (-246, 232.4737, -308.125) makes body 381 at (-246, 232.4737, -323.2812) makes body 380 at (-246, 232.4737, -5) in component "Обшивка-Доски-Вертикально"
delete_body "RemoveBody30" bodies 380 in component "Обшивка-Доски-Вертикально"
delete_body "RemoveBody31" bodies 383 in component "Обшивка-Доски-Вертикально"
delete_body "RemoveBody32" bodies 384 in component "Обшивка-Доски-Вертикально"
delete_body "RemoveBody33" bodies 396 in component "Обшивка-Доски-Вертикально"
delete_body "RemoveBody34" bodies 397 in component "Обшивка-Доски-Вертикально"
delete_body "RemoveBody35" bodies 398 in component "Обшивка-Доски-Вертикально"
delete_body "RemoveBody36" bodies 392 in component "Обшивка-Доски-Вертикально"
delete_body "RemoveBody37" bodies 386 in component "Обшивка-Доски-Вертикально"
delete_body "RemoveBody38" bodies 382 in component "Обшивка-Доски-Вертикально"
delete_body "RemoveBody39" bodies 388 in component "Обшивка-Доски-Вертикально"
delete_body "RemoveBody40" bodies 391 in component "Обшивка-Доски-Вертикально"
delete_body "RemoveBody41" bodies 390 in component "Обшивка-Доски-Вертикально"
delete_body "RemoveBody42" bodies 395 in component "Обшивка-Доски-Вертикально"
delete_body "RemoveBody43" bodies 387 in component "Обшивка-Доски-Вертикально"
delete_body "RemoveBody44" bodies 389 in component "Обшивка-Доски-Вертикально"
delete_body "RemoveBody45" bodies 393 in component "Обшивка-Доски-Вертикально"
delete_body "RemoveBody46" bodies 385 in component "Обшивка-Доски-Вертикально"
delete_body "RemoveBody47" bodies 394 in component "Обшивка-Доски-Вертикально"
delete_body "RemoveBody48" bodies 399 in component "Обшивка-Доски-Вертикально"
delete_body "RemoveBody49" bodies 381 in component "Обшивка-Доски-Вертикально"
delete_body "RemoveBody50" bodies 411 in component "Обшивка-Доски-Вертикально"
delete_body "RemoveBody51" bodies 404 in component "Обшивка-Доски-Вертикально"
delete_body "RemoveBody52" bodies 402 in component "Обшивка-Доски-Вертикально"
delete_body "RemoveBody53" bodies 407 in component "Обшивка-Доски-Вертикально"
delete_body "RemoveBody54" bodies 405 in component "Обшивка-Доски-Вертикально"
delete_body "RemoveBody55" bodies 403 in component "Обшивка-Доски-Вертикально"
delete_body "RemoveBody56" bodies 412 in component "Обшивка-Доски-Вертикально"
delete_body "RemoveBody57" bodies 406 in component "Обшивка-Доски-Вертикально"
delete_body "RemoveBody58" bodies 401 in component "Обшивка-Доски-Вертикально"
delete_body "RemoveBody59" bodies 409 in component "Обшивка-Доски-Вертикально"
delete_body "RemoveBody60" bodies 408 in component "Обшивка-Доски-Вертикально"
delete_body "RemoveBody61" bodies 400 in component "Обшивка-Доски-Вертикально"
delete_body "RemoveBody62" bodies 410 in component "Обшивка-Доски-Вертикально"
sketch "Sketch1 (12)" plane through (5, 0, 0) normal (1, 0, 0) x (0, 0, -1) in component "Двери"
  line L0 (255, 245.7192) -> (255, 20)
  line L1 (255, 20) -> (260, 20)
  line L2 (260, 20) -> (260, 245.7192)
  line L3 (260, 245.7192) -> (255, 245.7192)
  line L4 (125, 210.0714) -> (250, 210.0714)
  line L5 (250, 210.0714) -> (250, 20)
  line L6 (250, 20) -> (125, 20)
  line L7 (125, 20) -> (125, 210.0714)
  line L8 (187.5, 210.0714) -> (187.5, 20)
  line L9 (245, 25) -> (130, 25)
  line L10 (130, 20) -> (130, 210.0714)
  line L11 (130, 205.0714) -> (245, 205.0714)
  line L12 (245, 210.0714) -> (245, 20)
  line L13 (182.5, 210.0714) -> (182.5, 20)
  line L14 (192.5, 210.0714) -> (192.5, 20)
  line L15 (130, 115.0357) -> (182.5, 115.0357)
  line L16 (245, 115.0357) -> (192.5, 115.0357)
  line L17 (130, 110.0357) -> (182.5, 110.0357)
  line L18 (245, 110.0357) -> (192.5, 110.0357)
  point P0 (125, 20)
  point P1 (125, 210.0714)
  point P2 (250, 210.0714)
  point P3 (250, 20)
  point P4 (187.5, 210.0714)
  point P5 (187.5, 20)
  point P6 (130, 115.0357)
  point P7 (245, 115.0357)
  dimension "d333" = 5
  dimension "d334" = -5
  dimension "d335" = 5
  dimension "d336" = -5
  constraint horizontal L4
  constraint vertical L5
  constraint horizontal L6
  constraint vertical L7
  constraint coincident P3 L5.end
  constraint coincident P1 L4.start
  constraint midpoint L4 P4
  constraint midpoint L6 P5
  constraint coincident P4 L8.start
  constraint coincident P5 L8.end
  constraint coincident L4 L10.end
  constraint coincident L11.start L10
  constraint coincident L9.end L10
  constraint coincident L9.start L12
  constraint coincident L4 L12.start
  constraint coincident L11.end L12
  constraint midpoint L10 P6
  constraint midpoint L12 P7
  constraint coincident P6 L15.start
  constraint midpoint L13 L15.end
  constraint perpendicular L13 L15
  constraint coincident P7 L16.start
  constraint midpoint L14 L16.end
  constraint perpendicular L14 L16
extrude "Extrude1'''''''''''" add sketch "Sketch1 (12)" against normal blind 5 separate body contours L4 L6 L7 L10 | L4 L10 L11 L13 | L4 L8 L11 L13 | L6 L9 L10 L13 | L8 L9 L11 L13 | L10 L13 L15 L17 | L6 L8 L9 L13 makes body 413 in component "ДверьЛев"
extrude "Extrude1''''''''''''" add sketch "Sketch1 (12)" against normal blind 5 separate body contours L4 L8 L11 L14 | L4 L11 L12 L14 | L8 L9 L11 L14 | L6 L8 L9 L14 | L4 L5 L6 L12 | L6 L9 L12 L14 | L12 L14 L16 L18 makes body 414 in component "ДверьПрав"
combine "Combine1''''" [suppressed] in component "Обшивка-Плиты"
component "Обвязка" placed x (1, 0, 0) y (0, 1, 0) z (0, 0, 1) at (0, 0, 0)
component "Фундамент" placed x (1, 0, 0) y (0, 1, 0) z (0, 0, 1) at (0, 0, 0)
component "ЛицеваяСтена" placed x (1, 0, 0) y (0, 1, 0) z (0, 0, 1) at (0, 0, 0)
component "ЗадняяСтена" placed x (1, 0, 0) y (0, 1, 0) z (0, 0, 1) at (0, 0, 0)
component "БоковаяСтена" placed x (1, 0, 0) y (0, 1, 0) z (0, 0, 1) at (0, 0, 0)
component "БоковаяСтена(Mirror)" placed x (1, 0, 0) y (0, 1, 0) z (0, 0, 1) at (0, 0, -500)
component "Лаги" placed x (1, 0, 0) y (0, 1, 0) z (0, 0, 1) at (0, 0, 0)
component "Стропила" placed x (1, 0, 0) y (0, 1, 0) z (0, 0, 1) at (0, 0, 0)
component "Пол" placed x (1, 0, 0) y (0, 1, 0) z (0, 0, 1) at (0, 0, 0)
component "Обрешетка" placed x (1, 0, 0) y (0, 1, 0) z (0, 0, 1) at (0, 0, 0)
component "Крыша" placed x (1, 0, 0) y (0, 1, 0) z (0, 0, 1) at (0, 0, 0)
component "Обшивка-Плиты" placed x (1, 0, 0) y (0, 1, 0) z (0, 0, 1) at (0, 0, 0)
component "Обшивка-Доски" placed x (1, 0, 0) y (0, 1, 0) z (0, 0, 1) at (0, 0, 0)
component "Обшивка-Доски-Вертикально" placed x (1, 0, 0) y (0, 1, 0) z (0, 0, 1) at (0, 0, 0)
component "Двери" placed x (1, 0, 0) y (0, 1, 0) z (0, 0, 1) at (0, 0, 0)
component "ДверьЛев" placed x (0.835001, 0, 0.550249) y (0, 1, 0) z (-0.550249, 0, 0.835001) at (-67.9561, 0, -23.3761) in component "Двери"
component "ДверьПрав" placed x (0.602662, 0, -0.797996) y (0, 1, 0) z (0.797996, 0, 0.602662) at (201.4858, 0, -95.3444) in component "Двери"
equation "d173 = 250 mm + 2.5 mm"
